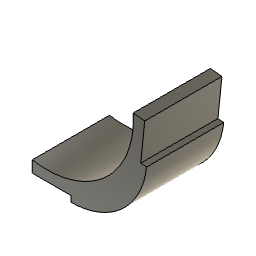
corner_frontbottom v1 (Autodesk Fusion 360 design; units mm, degrees)
Autodesk Fusion 360 part; units mm, degrees
sketch "Front, Bottom corner" plane through (0, 0, 0) normal (0, 1, 0) x (1, 0, 0)
  circle A0 centre (2038.212, 2.1526) radius 25 construction
  line L0 (2073.9927, -100.7451) -> (2060.9213, 25.5804) construction
  line L1 (1557.274, 27.1526) -> (2059.178, 27.1526) construction
  line L2 (2038.212, 27.1526) -> (2038.212, 25.2476)
  line L3 (2038.212, 25.2476) -> (2025.512, 25.2476)
  line L4 (2025.512, 25.2476) -> (2025.512, 21.4376)
  line L5 (2063.0792, 4.7257) -> (2061.1843, 4.5296)
  line L6 (2061.1843, 4.5296) -> (2062.4914, -8.1029)
  line L7 (2062.4914, -8.1029) -> (2058.7017, -8.4951)
  arc A1 (2063.0792, 4.7257) -> (2038.212, 27.1526) centre (2038.212, 2.1526) ccw
  line L8 (2038.212, 2.1526) -> (2054.9552, 20.7177) construction
  arc A2 (2058.7017, -8.4951) -> (2025.512, 21.4376) centre (2030.3296, -6.5875) ccw
  point P0 (2049.3741, 14.5294)
extrude "Extrude1" add sketch "Front, Bottom corner" along normal blind 25.4
